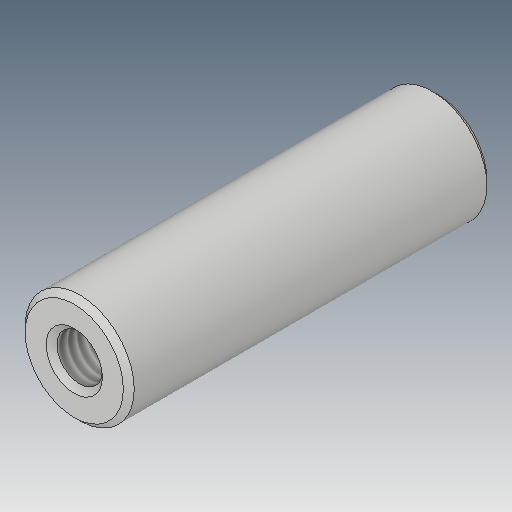
# Autodesk Inventor part: p9ALshaft
Saved by Autodesk Inventor 2019.4 (Build 234330000, 330)
## iProperties
Created: 2019-06-13
Part Number: p9ALshaft
Material: アルミニウム 2014-T4
Document SubType Name: Modeling
Designer: AzLIer
Density: 2.8 g/cm^3
Appearance: サテン
Mass: 1.30174 g
Surface Area: 5.71416 cm^2
Volume: 0.464909 cm^3
Author: AzLIer
Autodesk Inventor part; units mm, degrees
ref_plane "YZ Plane" through (0, 0, 0) normal (1, 0, 0) x (0, 1, 0)
ref_plane "XZ Plane" through (0, 0, 0) normal (0, 1, 0) x (-1, 0, 0)
ref_plane "XY Plane" through (0, 0, 0) normal (0, 0, 1) x (1, 0, 0)
sketch "スケッチ1" plane through (0, 0, 0) normal (0, 0, 1) x (1, 0, 0)
  circle A0 centre (0, 0) radius 3
  circle A1 centre (0, 0) radius 1.25
  dimension "d0" = 6
  dimension "d1" = 2.5
  constraints: 2 centre point, 2 coincident
  measures "d0" diameter of A0
  measures "d1" diameter of A1
extrude "押し出し1" add sketch "スケッチ1" along normal blind 20
chamfer "面取り1" distance 0.3 angle 45 4 edges at (-3, 0, 20) (-1.25, 0, 20) (-3, 0, 0) (-1.25, 0, 0)
thread "ねじ1" size "M3x0.5" class "6H" standard "ANSI Metric M Profile" full length
